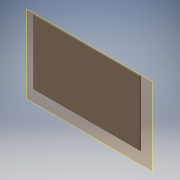
# Autodesk Inventor part: Zwischenplatt
Saved by Autodesk Inventor 2016 SP2 (Build 200236200, 236)
## iProperties
Created: 2018-06-21
Part Number: Zwischenplatt
Material: Generisch
Document SubType Name: Modeling
Designer: Nils
Density: 1 g/cm^3
Appearance: Vorgabe
Author: Nils
Autodesk Inventor part; units mm, degrees
ref_plane "YZ Plane" through (0, 0, 0) normal (1, 0, 0) x (0, 1, 0)
ref_plane "XZ Plane" through (0, 0, 0) normal (0, 1, 0) x (-1, 0, 0)
ref_plane "XY Plane" through (0, 0, 0) normal (0, 0, 1) x (1, 0, 0)
ref_plane "Arbeitsebene1" through (388.145, -180.4216, 157.1697) normal (0, -1, 0) x (0, 0, -1)
sketch "Skizze2" plane through (388.145, -180.4216, 157.1697) normal (0, -1, 0) x (0, 0, -1)
  line L0 (-139.4, -160.75) -> (-11.25, -160.75) construction
  line L1 (-139.4, -160.75) -> (-11.25, -160.75) construction
  line L2 (-11.25, -8.75) -> (-139.4, -8.75) construction
  line L3 (-11.25, -160.75) -> (-11.25, -8.75) construction
  line L4 (-102.5, -160) -> (-102.5, -9.5) construction
  line L5 (-102.5, -160.65) -> (-11.35, -160.65)
  line L6 (-11.35, -160.65) -> (-11.35, -8.85)
  line L7 (-11.35, -8.85) -> (-102.5, -8.85)
  line L8 (-102.5, -8.85) -> (-102.5, -160.65)
  point P0 (157.1697, -388.145)
  dimension "d7" = 0.1
  dimension "d8" = 0.1
  dimension "d9" = 0.1
  constraints: 8 end point, 2 parallel, 1 collinear, 1 horizontal, 1 perpendicular
  measures "d7" distance between parallel lines of L2 L7
  measures "d8" distance between parallel lines of L6 L3
  measures "d9" distance between parallel lines of L0 L5
extrude "Extrusion2" add sketch "Skizze2" against normal blind 1.5
chamfer "Fase2" distance 0.75 angle 45 6 edges at (227.495, -178.9216, 214.0947) (227.495, -180.4216, 214.0947) (303.395, -178.9216, 168.5197) (303.395, -180.4216, 168.5197) (379.295, -178.9216, 214.0947) (379.295, -180.4216, 214.0947)
equation "\"d7\" = d8"
equation "\"d9\" = d8"
